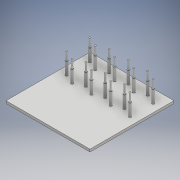
# Autodesk Inventor part: Palma
Saved by Autodesk Inventor 2018 (Build 220112000, 112)
## iProperties
Created: 2017-06-01
Part Number: Palma
Material: Genérico
Document SubType Name: Modeling
Designer: Vitor
Density: 1 g/cm^3
Appearance: Padrão
Author: Vitor
Autodesk Inventor part; units mm, degrees
ref_plane "YZ Plane" through (0, 0, 0) normal (1, 0, 0) x (0, 1, 0)
ref_plane "XZ Plane" through (0, 0, 0) normal (0, 1, 0) x (-1, 0, 0)
ref_plane "XY Plane" through (0, 0, 0) normal (0, 0, 1) x (1, 0, 0)
sketch "Esboço1" plane through (0, 0, 0) normal (0, 0, 1) x (1, 0, 0)
  line L0 (0, 0) -> (100, 0)
  line L1 (100, 0) -> (100, -100)
  line L2 (100, -100) -> (0, -100)
  line L3 (0, -100) -> (0, 0)
  dimension "d0" = 100
  dimension "d1" = 100
  constraints: 8 end point, 2 parallel, 1 horizontal, 1 perpendicular
  measures "d0" distance of L1.end L2.end
  measures "d1" distance of L0.end L1.end
extrude "Extrusão1" add sketch "Esboço1" along normal blind 3
sketch "Esboço2" plane through (0, 0, 3) normal (0, 0, 1) x (1, 0, 0)
  line L0 (0, 0) -> (0, -100) projected
  line L1 (0, 0) -> (9.75, 0)
  line L2 (100, 0) -> (0, 0) projected
  line L3 (9.75, 0) -> (9.75, -10)
  line L4 (9.75, 0) -> (21.25, 0)
  line L5 (21.25, 0) -> (32.75, 0)
  line L6 (32.75, 0) -> (44.25, 0)
  line L7 (44.25, 0) -> (55.75, 0)
  line L8 (55.75, 0) -> (67.25, 0)
  line L9 (67.25, 0) -> (78.75, 0)
  line L10 (78.75, 0) -> (90.25, 0)
  line L11 (90.25, 0) -> (100, 0)
  line L12 (21.25, 0) -> (21.25, -10)
  line L13 (9.75, -10) -> (9.75, -37.6)
  line L14 (9.75, -37.6) -> (21.25, -37.6)
  line L15 (21.25, -37.6) -> (32.75, -37.6)
  line L16 (32.75, -37.6) -> (44.25, -37.6)
  line L17 (44.25, -37.6) -> (55.75, -37.6)
  line L18 (55.75, -37.6) -> (67.25, -37.6)
  line L19 (67.25, -37.6) -> (78.75, -37.6)
  line L20 (78.75, -37.6) -> (90.25, -37.6)
  line L21 (90.25, -37.6) -> (90.25, -10)
  line L22 (90.25, -10) -> (78.75, -10)
  line L23 (78.75, -10) -> (67.25, -10)
  line L24 (67.25, -10) -> (55.75, -10)
  line L25 (55.75, -10) -> (44.25, -10)
  line L26 (44.25, -10) -> (32.75, -10)
  line L27 (32.75, -10) -> (21.25, -10)
  circle A0 centre (9.75, -10) radius 1.5
  circle A1 centre (9.75, -37.6) radius 1.5
  circle A2 centre (32.75, -10) radius 1.5
  circle A3 centre (55.75, -10) radius 1.5
  circle A4 centre (78.75, -10) radius 1.5
  circle A5 centre (78.75, -37.6) radius 1.5
  circle A6 centre (55.75, -37.6) radius 1.5
  circle A7 centre (32.75, -37.6) radius 1.5
  line L28 (21.25, -10) -> (21.25, -15)
  line L29 (21.25, -15) -> (44.25, -15)
  line L30 (44.25, -15) -> (67.25, -15)
  line L31 (67.25, -15) -> (90.25, -15)
  line L32 (21.25, -15) -> (21.25, -42.6)
  line L33 (21.25, -42.6) -> (44.25, -42.6)
  line L34 (44.25, -42.6) -> (67.25, -42.6)
  line L35 (67.25, -42.6) -> (90.25, -42.6)
  circle A8 centre (21.25, -42.6) radius 1.5
  circle A9 centre (44.25, -42.6) radius 1.5
  circle A10 centre (67.25, -42.6) radius 1.5
  circle A11 centre (90.25, -42.6) radius 1.5
  circle A12 centre (90.25, -15) radius 1.5
  circle A13 centre (44.25, -15) radius 1.5
  circle A14 centre (21.25, -15) radius 1.5
  circle A15 centre (67.25, -15) radius 1.5
  dimension "d4" = 9.75
  dimension "d5" = 10
  dimension "d7" = 11.5
  dimension "d8" = 11.5
  dimension "d9" = 11.5
  dimension "d10" = 11.5
  dimension "d11" = 11.5
  dimension "d12" = 11.5
  dimension "d13" = 11.5
  dimension "d14" = 27.6
  dimension "d16" = 3
  dimension "d17" = 3
  dimension "d19" = 3
  dimension "d21" = 3
  dimension "d23" = 3
  dimension "d26" = 3
  dimension "d28" = 3
  dimension "d30" = 3
  dimension "d60" = 5
  dimension "d61" = 27.6
  dimension "d62" = 3
  dimension "d63" = 3
  dimension "d64" = 3
  dimension "d65" = 3
  dimension "d66" = 3
  dimension "d68" = 3
  dimension "d69" = 3
  dimension "d70" = 3
  constraints: 68 end point, 17 coincident, 16 centre point, 16 point on line, 5 perpendicular, 3 vertical, 2 horizontal, 1 collinear, 9 other
  measures "d4" distance of L0.start L1.end
  measures "d5" distance of L1.end L3.end
  measures "d7" distance of L1.end L4.end
  measures "d8" distance of L4.end L5.end
  measures "d9" distance of L5.end L6.end
  measures "d10" distance of L6.end L7.end
  measures "d11" distance of L7.end L8.end
  measures "d12" distance of L8.end L9.end
  measures "d13" distance of L9.end L10.end
  measures "d14" distance of L13.start L13.end
  measures "d16" diameter of A0
  measures "d17" diameter of A1
  measures "d19" diameter of A2
  measures "d21" diameter of A3
  measures "d23" diameter of A4
  measures "d26" diameter of A5
  measures "d28" diameter of A6
  measures "d30" diameter of A7
  measures "d60" distance of L12.end L28.end
  measures "d61" distance of L28.end L32.end
  measures "d62" diameter of A8
  measures "d63" diameter of A9
  measures "d64" diameter of A10
  measures "d65" diameter of A11
  measures "d66" diameter of A12
  measures "d68" diameter of A13
  measures "d69" diameter of A14
  measures "d70" diameter of A15
extrude "Extrusão4" add sketch "Esboço2" along normal blind 15 contours A0 L13 L3 | L3 L13 A0 | A2 L26 L27 | L27 L26 A2 | A14 L29 L28 | L28 L32 A14 | L29 A14 L32 | A1 L14 L13 | L13 L14 A1 | A13 L30 L29 | L29 L30 A13 | A3 L24 L25 | L25 L24 A3 | A7 L16 L15 | L15 L16 A7 | A15 L31 L30 | L30 L31 A15 | A4 L22 L23 | L23 L22 A4 | A12 L21 L31 | L31 L21 A12 | A6 L18 L17 | L17 L18 A6 | L21 A12 | A5 L19 L20 | L20 L19 A5 | A8 L33 L32 | L32 L33 A8 | A9 L34 L33 | L33 L34 A9 | A10 L35 L34 | L34 L35 A10 | A11
sketch "Esboço4" plane through (9.75, -10, 18) normal (0, 0, 1) x (1, 0, 0)
  line L0 (0, 0) -> (11.5, 0)
  circle A0 centre (23, 0) radius 1.5 projected
  line L1 (11.5, 0) -> (23, 0)
  line L2 (23, 0) -> (34.5, 0)
  circle A1 centre (46, 0) radius 1.5 projected
  line L3 (34.5, 0) -> (46, 0)
  line L4 (46, 0) -> (57.5, 0)
  line L5 (57.5, 0) -> (69, 0)
  line L6 (69, 0) -> (80.5, 0)
  line L7 (80.5, 0) -> (80.5, -27.6)
  circle A2 centre (69, -27.6) radius 1.5 projected
  line L8 (80.5, -27.6) -> (69, -27.6)
  line L9 (69, -27.6) -> (57.5, -27.6)
  line L10 (57.5, -27.6) -> (46, -27.6)
  line L11 (46, -27.6) -> (34.5, -27.6)
  line L12 (34.5, -27.6) -> (23, -27.6)
  line L13 (23, -27.6) -> (11.5, -27.6)
  line L14 (11.5, -27.6) -> (0, -27.6)
  line L15 (0, -27.6) -> (0, -32.6)
  line L16 (0, -32.6) -> (11.5, -32.6)
  line L17 (11.5, -32.6) -> (34.5, -32.6)
  line L18 (34.5, -32.6) -> (57.5, -32.6)
  line L19 (57.5, -32.6) -> (80.5, -32.6)
  circle A3 centre (11.5, -5) radius 1.5 projected
  line L20 (11.5, 0) -> (11.5, -5)
  line L21 (11.5, -5) -> (34.5, -5)
  circle A4 centre (57.5, -5) radius 1.5 projected
  line L22 (34.5, -5) -> (57.5, -5)
  line L23 (57.5, -5) -> (80.5, -5)
  circle A5 centre (11.5, -5) radius 0.95
  circle A6 centre (23, 0) radius 0.95
  circle A7 centre (0, 0) radius 1.5 projected
  circle A8 centre (34.5, -5) radius 1.5 projected
  circle A9 centre (34.5, -5) radius 0.95
  circle A10 centre (46, 0) radius 0.95
  circle A11 centre (57.5, -5) radius 0.95
  circle A12 centre (69, 0) radius 1.5 projected
  circle A13 centre (69, 0) radius 0.95
  circle A14 centre (80.5, -5) radius 0.95
  circle A15 centre (0, -27.6) radius 1.5 projected
  circle A16 centre (0, -27.6) radius 0.95
  circle A17 centre (11.5, -32.6) radius 0.95
  circle A18 centre (23, -27.6) radius 0.95
  circle A19 centre (34.5, -32.6) radius 0.95
  circle A20 centre (46, -27.6) radius 1.5 projected
  circle A21 centre (46, -27.6) radius 0.95
  circle A22 centre (57.5, -32.6) radius 0.95
  circle A23 centre (69, -27.6) radius 0.95
  circle A24 centre (80.5, -32.6) radius 0.95
  circle A25 centre (0, 0) radius 0.95
  point P0 (-9.75, 10)
  dimension "d73" = 11.5
  dimension "d74" = 11.5
  dimension "d75" = 11.5
  dimension "d76" = 11.5
  dimension "d77" = 11.5
  dimension "d78" = 11.5
  dimension "d79" = 11.5
  dimension "d80" = 27.6
  dimension "d81" = 5
  dimension "d82" = 1.9
  dimension "d83" = 1.9
  dimension "d85" = 1.9
  dimension "d86" = 1.9
  dimension "d87" = 1.9
  dimension "d88" = 1.9
  dimension "d89" = 1.9
  dimension "d90" = 1.9
  dimension "d91" = 1.9
  dimension "d92" = 1.9
  dimension "d93" = 1.9
  dimension "d94" = 1.9
  dimension "d95" = 1.9
  dimension "d96" = 1.9
  dimension "d97" = 1.9
  dimension "d98" = 1.9
  constraints: 48 end point, 16 centre point, 16 coincident, 16 point on line, 4 perpendicular, 2 collinear, 1 horizontal
  measures "d73" distance of L0.start L0.end
  measures "d74" distance of L0.end L1.end
  measures "d75" distance of L1.end L2.end
  measures "d76" distance of L2.end L3.end
  measures "d77" distance of L3.end L4.end
  measures "d78" distance of L4.end L5.end
  measures "d79" distance of L5.end L6.end
  measures "d80" distance of L6.end L7.end
  measures "d81" distance of L14.end L15.end
  measures "d82" diameter of A5
  measures "d83" diameter of A6
  measures "d85" diameter of A9
  measures "d86" diameter of A10
  measures "d87" diameter of A11
  measures "d88" diameter of A13
  measures "d89" diameter of A14
  measures "d90" diameter of A16
  measures "d91" diameter of A17
  measures "d92" diameter of A18
  measures "d93" diameter of A19
  measures "d94" diameter of A21
  measures "d95" diameter of A22
  measures "d96" diameter of A23
  measures "d97" diameter of A24
  measures "d98" diameter of A25
extrude "Extrusão5" add sketch "Esboço4" along normal blind 10 contours A6 L1 L2 | L2 L1 A6 | A10 L4 L3 | L3 L4 A10 | A5 L21 L20 | L20 L21 A5 | A9 L22 L21 | L21 L22 A9 | A13 L6 L5 | L5 L6 A13 | A11 L23 L22 | L22 L23 A11 | A14 L7 | L7 L23 A14 | L23 L7 A14 | A23 L9 L8 | L8 L9 A23 | A21 L11 L10 | L10 L11 A21 | A18 L13 L12 | L12 L13 A18 | A16 L15 L14 | L14 L15 A16 | A17 L17 L16 | L16 L17 A17 | A19 L18 L17 | L17 L18 A19 | A22 L19 L18 | L18 L19 A22 | A24 | A25
